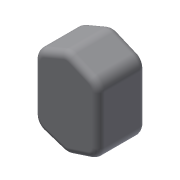
# Autodesk Inventor part: body
Saved by Autodesk Inventor 2014 SP1 (Build 180222100, 222)
## iProperties
Created: 2015-02-04
Part Number: body
Material: Generic
Document SubType Name: Modeling
Designer: Simen
Density: 1 g/cm^3
Appearance: Default
Author: Simen
Autodesk Inventor part; units mm, degrees
ref_plane "YZ Plane" through (0, 0, 0) normal (1, 0, 0) x (0, 1, 0)
ref_plane "XZ Plane" through (0, 0, 0) normal (0, 1, 0) x (-1, 0, 0)
ref_plane "XY Plane" through (0, 0, 0) normal (0, 0, 1) x (1, 0, 0)
sketch "Sketch1" plane through (0, 0, 0) normal (0, 1, 0) x (-1, 0, 0)
  line L0 (-8.4597, -4.2821) -> (491.5403, -4.2821)
  line L1 (491.5403, -4.2821) -> (491.5403, 692.7179)
  line L2 (491.5403, 692.7179) -> (-8.4597, 692.7179)
  line L3 (-8.4597, 692.7179) -> (-8.4597, -4.2821)
  point P0 (0, 0)
  dimension "d0" = 500
  dimension "d1" = 697
  constraints: 8 end point, 2 parallel, 1 horizontal, 1 perpendicular
  measures "d0" distance of L2.end L1.end
  measures "d1" distance of L1.end L0.end
extrude "Extrusion1" add sketch "Sketch1" along normal blind 372
sketch "Sketch2" plane through (0, 372, 0) normal (0, 1, 0) x (1, 0, 0)
  line L0 (8.4597, 4.2821) -> (-491.5403, 4.2821) projected
  line L1 (-491.5403, 4.2821) -> (-491.5403, -692.7179) projected
  line L2 (-491.5403, -692.7179) -> (8.4597, -692.7179) projected
  line L3 (8.4597, -692.7179) -> (8.4597, 4.2821) projected
  line L4 (-241.5403, 4.2821) -> (-491.5403, -77.8084)
  line L5 (-241.5403, 4.2821) -> (8.4597, -77.8084)
  line L6 (8.4597, -586.8499) -> (-241.5403, -692.7179)
  line L7 (-241.5403, -692.7179) -> (-491.5403, -586.8499)
  point P0 (0, 0)
  constraints: 8 end point, 4 point on line, 2 midpoint
extrude "Extrusion2" cut sketch "Sketch2" against normal blind 400 contours L3 L5 L0 | L4 L1 L0 | L3 L2 L6 | L7 L2 L1
fillet "Fillet1" radius 100 6 edges at (-241.5403, 186, 692.7179) (8.4597, 186, 586.8499) (-491.5403, 186, 586.8499) (8.4597, 186, 77.8084) (-241.5403, 186, -4.2821) (-491.5403, 186, 77.8084)
fillet "Fillet2" radius 50 24 edges at (-10.5472, 372, 91.5727) (-135.3429, 372, 30.5891) (-241.5403, 372, 0.971) (-347.7376, 372, 30.5891) (-472.5333, 372, 91.5727) (-491.5403, 372, 335.4127) (-474.9054, 372, 575.8293) (-355.5351, 372, 644.4443) (-241.5403, 372, 684.121) (-127.5454, 372, 644.4443) (-8.1751, 372, 575.8293) (8.4597, 372, 335.4127) (-10.5472, 0, 91.5727) (-135.3429, 0, 30.5891) (-241.5403, 0, 0.971) (-347.7376, 0, 30.5891) (-472.5333, 0, 91.5727) (-491.5403, 0, 335.4127) (-474.9054, 0, 575.8293) (-355.5351, 0, 644.4443) (-241.5403, 0, 684.121) (-127.5454, 0, 644.4443) (-8.1751, 0, 575.8293) (8.4597, 0, 335.4127)
body "Solid1"
